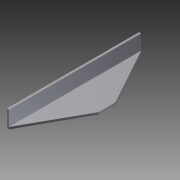
# Autodesk Inventor part: 8 ball mount L
Saved by Autodesk Inventor 2012 (Build 160160000, 160)
## iProperties
Created: 2013-10-10
Part Number: 8 ball mount L
Material: Default
Document SubType Name: Modeling
Designer: Bryce
Density: 1 g/cm^3
Author: Bryce
Autodesk Inventor part; units mm, degrees
ref_plane "YZ Plane" through (0, 0, 0) normal (1, 0, 0) x (0, 1, 0)
ref_plane "XZ Plane" through (0, 0, 0) normal (0, 1, 0) x (-1, 0, 0)
ref_plane "XY Plane" through (0, 0, 0) normal (0, 0, 1) x (1, 0, 0)
sketch "Sketch1" plane through (0, 0, 0) normal (0, 0, 1) x (1, 0, 0)
  line L0 (0, 0) -> (50.8, 0)
  line L1 (50.8, 0) -> (50.8, 3.175)
  line L2 (3.175, 25.4) -> (0, 25.4)
  line L3 (0, 25.4) -> (0, 0)
  line L4 (3.175, 25.4) -> (3.175, 3.175)
  line L5 (3.175, 3.175) -> (50.8, 3.175)
  dimension "d0" = 50.8
  dimension "d1" = 25.4
  dimension "d2" = 3.175
  dimension "d3" = 3.175
  constraints: 12 end point, 2 parallel, 1 horizontal, 1 perpendicular
  measures "d0" distance of L0.start L0.end
  measures "d1" distance of L2.end L0.start
  measures "d2" distance between parallel lines of L3 L4
  measures "d3" distance between parallel lines of L0 L5
extrude "Extrusion1" add sketch "Sketch1" along normal blind 196.85
sketch "Sketch2" plane through (0, 0, 0) normal (0, -1, 0) x (1, 0, 0)
  line L0 (50.8, 196.85) -> (0, 196.85) projected
  line L1 (50.8, 0) -> (50.8, 196.85) projected
  line L2 (3.175, 0) -> (3.175, 196.85) projected
  line L3 (3.175, 111.125) -> (50.8, 111.125)
  line L4 (50.8, 111.125) -> (50.8, 85.725)
  line L5 (50.8, 85.725) -> (3.175, 85.725)
  line L6 (3.175, 85.725) -> (3.175, 111.125)
  line L7 (0, 0) -> (50.8, 0) projected
  line L8 (50.8, 85.725) -> (3.175, 0)
  line L9 (50.8, 111.125) -> (3.175, 196.85)
  dimension "d18" = 25.4
  dimension "d19" = 85.725
  dimension "d20" = 85.725
  constraints: 12 end point, 2 parallel, 2 point on line, 1 horizontal, 1 perpendicular
  measures "d18" distance of L3.end L4.end
  measures "d19" distance between parallel lines of L0 L3
  measures "d20" distance between parallel lines of L7 L5
extrude "Extrusion4" cut sketch "Sketch2" against normal through all contours L1 L9 L0 | L1 L7 L8
equation "\"d2\" = d3"
equation "\"d19\" = d20"
body "Solid1"
